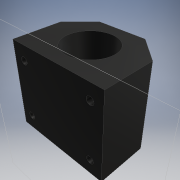
# Autodesk Inventor part: BracketLineal
Saved by Autodesk Inventor 2018 (Build 220112000, 112)
## iProperties
Created: 2018-01-02
Part Number: BracketLineal
Material: Plástico ABS
Document SubType Name: Modeling
Designer: Carlos
Density: 1.06 g/cm^3
Appearance: Suave - Blanco
Author: Carlos
Autodesk Inventor part; units mm, degrees
ref_plane "YZ Plane" through (0, 0, 0) normal (1, 0, 0) x (0, 1, 0)
ref_plane "XZ Plane" through (0, 0, 0) normal (0, 1, 0) x (-1, 0, 0)
ref_plane "XY Plane" through (0, 0, 0) normal (0, 0, 1) x (1, 0, 0)
sketch "Boceto2" plane through (0, 0, 0) normal (0, 0, 1) x (1, 0, 0)
  line L0 (-20, -10) -> (20, -10)
  line L1 (20, -10) -> (20, 10)
  line L2 (20, 10) -> (-20, 10)
  line L3 (-20, 10) -> (-20, -10)
  line L4 (-20, -10) -> (20, 10) construction
  line L5 (20, -10) -> (-20, 10) construction
  line L6 (-20, 10) -> (-10, 20)
  line L7 (10, 20) -> (20, 10)
  line L8 (-10, 20) -> (10, 20)
  point P0 (0, 0)
  dimension "d0" = 20
  dimension "d1" = 40
  dimension "d2" = 10
  dimension "d3" = 10
  dimension "d4" = 10
  constraints: 18 end point, 2 horizontal, 2 midpoint, 2 parallel, 1 perpendicular
  measures "d0" distance of L0.end L1.end
  measures "d1" distance of L1.end L2.end
  measures "d2" horizontal distance of L7.start L1.end
  measures "d3" horizontal distance of L6.end L2.end
  measures "d4" distance between parallel lines of L2 L8
extrude "Extrusión1" add sketch "Boceto2" along normal blind 35
sketch "Boceto3" plane through (0, 0, 35) normal (0, 0, 1) x (1, 0, 0)
  circle A0 centre (0, 5) radius 10
  line L0 (-20, -10) -> (20, -10) projected
  point P0 (0, 0)
  dimension "d7" = 20
  dimension "d8" = 15
  constraints: 1 centre point
  measures "d7" diameter of A0
  measures "d8" distance from line of L0 A0.centre
hole "Agujero1" at (0, 5, 35) direction (0, 0, -1) diameter 20 depth 35 tip angle 118
sketch "Boceto4" plane through (-20, -10, 0) normal (0, -1, 0) x (1, 0, 0)
  line L0 (5, 6) -> (35, 6)
  line L1 (35, 6) -> (35, 29)
  line L2 (35, 29) -> (5, 29)
  line L3 (5, 29) -> (5, 6)
  line L4 (5, 6) -> (35, 29) construction
  line L5 (35, 6) -> (5, 29) construction
  line L6 (40, 0) -> (40, 35) projected
  line L7 (30, 0) -> (30, 35) projected
  line L8 (0, 0) -> (0, 35) projected
  line L9 (0, 35) -> (40, 35) projected
  line L10 (0, 0) -> (40, 0) projected
  point P0 (20, 0)
  point P1 (20, 17.5)
  dimension "d16" = 23
  dimension "d17" = 5
  dimension "d18" = 10
  dimension "d19" = 5
  dimension "d20" = 30
  dimension "d30" = 17.5
  dimension "d31" = 35
  constraints: 12 end point, 2 midpoint, 2 parallel, 1 horizontal, 1 perpendicular
  measures "d16" distance of L0.end L1.end
  measures "d17" distance between parallel lines of L6 L1
  measures "d18" distance between parallel lines of L6 L7
  measures "d19" distance between parallel lines of L8 L3
  measures "d20" distance of L1.end L2.end
  measures "d30" distance from line of L9 point (20, 17.5)
  measures "d31" distance between parallel lines of L9 L10
hole "Agujero2" at (-15, -10, 29) at (15, -10, 29) at (15, -10, 6) at (-15, -10, 6) direction (0, 1, 0) diameter 3 depth 35 tip angle 118
sketch "Boceto6" plane through (-10, 20, 0) normal (0, 1, 0) x (1, 0, 0)
  line L0 (-5, -29) -> (25, -29)
  line L1 (25, -29) -> (25, -6)
  line L2 (25, -6) -> (-5, -6)
  line L3 (-5, -6) -> (-5, -29)
  line L4 (-5, -29) -> (25, -6) construction
  line L5 (25, -29) -> (-5, -6) construction
  line L6 (20, 0) -> (0, 0) projected
  point P0 (10, 0)
  point P1 (10, -17.5)
  dimension "d32" = 17.5
  dimension "d33" = 30
  dimension "d34" = 23
  constraints: 12 end point, 2 midpoint, 2 parallel, 1 horizontal, 1 perpendicular
  measures "d32" distance from line of L6 point (10, -17.5)
  measures "d33" distance of L1.end L2.end
  measures "d34" distance of L0.end L1.end
hole "Agujero3" at (15, 20, 29) at (-15, 20, 29) at (-15, 20, 6) at (15, 20, 6) direction (0, -1, 0) diameter 5 depth 10 tip angle 118
